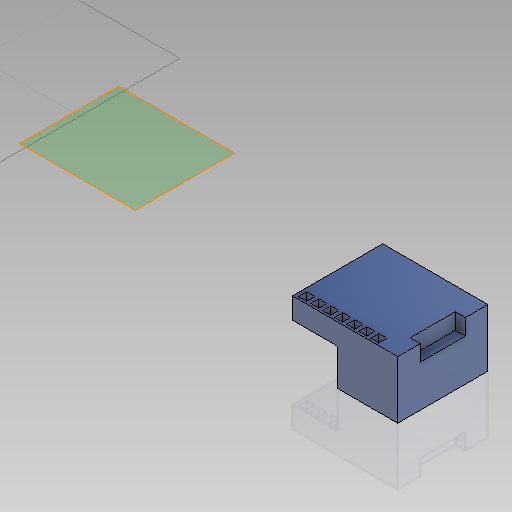
# Autodesk Inventor part: ЛЦМК0000002.00.00.00.00.04
Saved by Autodesk Inventor 2021.2 (Build 252289000, 289)
## iProperties
Created: 2025-10-23
Part Number: ЛЦМК0000002.00.00.00.00.04
Material: Типовые
Document SubType Name: Modeling
Designer: Захаров
Density: 1 g/cm^3
Appearance: С вкраплениями — сатинированная — синяя
Author: Захаров
Autodesk Inventor part; units mm, degrees
ref_plane "YZ Plane" through (0, 0, 0) normal (1, 0, 0) x (0, 1, 0)
ref_plane "XZ Plane" through (0, 0, 0) normal (0, 1, 0) x (-1, 0, 0)
ref_plane "XY Plane" through (0, 0, 0) normal (0, 0, 1) x (1, 0, 0)
ref_plane "РабПлоскость1" through (61.75, -2.8, -7.7) normal (0, -1, 0) x (1, 0, 0)
sketch "Эскиз1" plane through (61.75, -2.8, -7.7) normal (0, -1, 0) x (1, 0, 0)
  line L0 (49.15, 6.9) -> (47.55, 6.9) projected
  line L1 (47.55, 6.9) -> (47.55, 8.5) projected
  line L2 (47.55, 8.5) -> (49.15, 8.5) projected
  line L3 (49.15, 8.5) -> (49.15, 6.9) projected
  line L4 (44.35, 6.9) -> (42.75, 6.9) projected
  line L5 (42.75, 6.9) -> (42.75, 8.5) projected
  line L6 (42.75, 8.5) -> (44.35, 8.5) projected
  line L7 (44.35, 8.5) -> (44.35, 6.9) projected
  line L8 (53.95, 6.9) -> (52.35, 6.9) projected
  line L9 (52.35, 6.9) -> (52.35, 8.5) projected
  line L10 (52.35, 8.5) -> (53.95, 8.5) projected
  line L11 (53.95, 8.5) -> (53.95, 6.9) projected
  line L12 (51.55, 6.9) -> (49.95, 6.9) projected
  line L13 (49.95, 6.9) -> (49.95, 8.5) projected
  line L14 (49.95, 8.5) -> (51.55, 8.5) projected
  line L15 (51.55, 8.5) -> (51.55, 6.9) projected
  line L16 (56.35, 6.9) -> (54.75, 6.9) projected
  line L17 (54.75, 6.9) -> (54.75, 8.5) projected
  line L18 (54.75, 8.5) -> (56.35, 8.5) projected
  line L19 (56.35, 8.5) -> (56.35, 6.9) projected
  line L20 (46.75, 6.9) -> (45.15, 6.9) projected
  line L21 (45.15, 6.9) -> (45.15, 8.5) projected
  line L22 (45.15, 8.5) -> (46.75, 8.5) projected
  line L23 (46.75, 8.5) -> (46.75, 6.9) projected
  line L24 (58.75, 6.9) -> (57.15, 6.9) projected
  line L25 (57.15, 6.9) -> (57.15, 8.5) projected
  line L26 (57.15, 8.5) -> (58.75, 8.5) projected
  line L27 (58.75, 8.5) -> (58.75, 6.9) projected
  line L28 (61, 4.5) -> (63, 4.5) projected
  line L29 (63, 4.5) -> (63, 9) projected
  line L30 (63, 9) -> (42, 9) projected
  line L31 (42, 9) -> (42, -9) projected
  line L32 (42, -9) -> (63, -9) projected
  line L33 (63, -9) -> (63, -4.5) projected
  line L34 (63, -4.5) -> (61, -4.5) projected
  line L35 (61, -4.5) -> (61, 4.5) projected
  line L36 (47.55, -6.9) -> (49.15, -6.9) projected
  line L37 (49.15, -6.9) -> (49.15, -8.5) projected
  line L38 (49.15, -8.5) -> (47.55, -8.5) projected
  line L39 (47.55, -8.5) -> (47.55, -6.9) projected
  line L40 (42.75, -6.9) -> (44.35, -6.9) projected
  line L41 (44.35, -6.9) -> (44.35, -8.5) projected
  line L42 (44.35, -8.5) -> (42.75, -8.5) projected
  line L43 (42.75, -8.5) -> (42.75, -6.9) projected
  line L44 (52.35, -6.9) -> (53.95, -6.9) projected
  line L45 (53.95, -6.9) -> (53.95, -8.5) projected
  line L46 (53.95, -8.5) -> (52.35, -8.5) projected
  line L47 (52.35, -8.5) -> (52.35, -6.9) projected
  line L48 (49.95, -6.9) -> (51.55, -6.9) projected
  line L49 (51.55, -6.9) -> (51.55, -8.5) projected
  line L50 (51.55, -8.5) -> (49.95, -8.5) projected
  line L51 (49.95, -8.5) -> (49.95, -6.9) projected
  line L52 (54.75, -6.9) -> (56.35, -6.9) projected
  line L53 (56.35, -6.9) -> (56.35, -8.5) projected
  line L54 (56.35, -8.5) -> (54.75, -8.5) projected
  line L55 (54.75, -8.5) -> (54.75, -6.9) projected
  line L56 (45.15, -6.9) -> (46.75, -6.9) projected
  line L57 (46.75, -6.9) -> (46.75, -8.5) projected
  line L58 (46.75, -8.5) -> (45.15, -8.5) projected
  line L59 (45.15, -8.5) -> (45.15, -6.9) projected
  line L60 (57.15, -6.9) -> (58.75, -6.9) projected
  line L61 (58.75, -6.9) -> (58.75, -8.5) projected
  line L62 (58.75, -8.5) -> (57.15, -8.5) projected
  line L63 (57.15, -8.5) -> (57.15, -6.9) projected
  point P0 (-61.75, 7.7)
extrude "Выдавливание1" add sketch "Эскиз1" along normal blind 4.2 contours L35 L34 L33 L32 L31 L30 L29 L28 | L36 L37 L38 L39 | L40 L41 L42 L43 | L44 L45 L46 L47 | L48 L49 L50 L51 | L52 L53 L54 L55 | L56 L57 L58 L59 | L60 L61 L62 L63
sketch "Эскиз2" plane through (61.75, -7, -7.7) normal (0, -1, 0) x (1, 0, 0)
  line L0 (63, -9) -> (63, -4.5) projected
  line L1 (63, 9) -> (42, 9) projected
  line L2 (63, -9) -> (51, -9)
  line L3 (51, -9) -> (51, 9)
  line L4 (51, 9) -> (63, 9)
  line L5 (63, 9) -> (63, -9)
  point P0 (-61.75, 7.7)
  point P1 (63, -4.5)
  point P2 (63, 9)
  dimension "d2" = 12
  constraints: 8 end point, 2 parallel, 1 horizontal, 1 perpendicular, 1 point on line
  measures "d2" distance of L3.end L4.end
extrude "Выдавливание2" add sketch "Эскиз2" along normal blind 7.3
sketch "Эскиз3" plane through (61.75, -14.3, -7.7) normal (0, -1, 0) x (1, 0, 0)
  line L0 (47.55, 6.9) -> (49.15, 6.9) projected
  line L1 (49.15, 6.9) -> (49.15, 8.5) projected
  line L2 (49.15, 8.5) -> (47.55, 8.5) projected
  line L3 (47.55, 8.5) -> (47.55, 6.9) projected
  line L4 (42.75, 6.9) -> (44.35, 6.9) projected
  line L5 (44.35, 6.9) -> (44.35, 8.5) projected
  line L6 (44.35, 8.5) -> (42.75, 8.5) projected
  line L7 (42.75, 8.5) -> (42.75, 6.9) projected
  line L8 (52.35, 6.9) -> (53.95, 6.9) projected
  line L9 (53.95, 6.9) -> (53.95, 8.5) projected
  line L10 (53.95, 8.5) -> (52.35, 8.5) projected
  line L11 (52.35, 8.5) -> (52.35, 6.9) projected
  line L12 (49.95, 6.9) -> (51.55, 6.9) projected
  line L13 (51.55, 6.9) -> (51.55, 8.5) projected
  line L14 (51.55, 8.5) -> (49.95, 8.5) projected
  line L15 (49.95, 8.5) -> (49.95, 6.9) projected
  line L16 (54.75, 6.9) -> (56.35, 6.9) projected
  line L17 (56.35, 6.9) -> (56.35, 8.5) projected
  line L18 (56.35, 8.5) -> (54.75, 8.5) projected
  line L19 (54.75, 8.5) -> (54.75, 6.9) projected
  line L20 (45.15, 6.9) -> (46.75, 6.9) projected
  line L21 (46.75, 6.9) -> (46.75, 8.5) projected
  line L22 (46.75, 8.5) -> (45.15, 8.5) projected
  line L23 (45.15, 8.5) -> (45.15, 6.9) projected
  line L24 (57.15, 6.9) -> (58.75, 6.9) projected
  line L25 (58.75, 6.9) -> (58.75, 8.5) projected
  line L26 (58.75, 8.5) -> (57.15, 8.5) projected
  line L27 (57.15, 8.5) -> (57.15, 6.9) projected
  line L28 (63, 9) -> (42, 9) projected
  line L29 (63, -9) -> (63, 9) projected
  line L30 (42, -9) -> (63, -9) projected
  line L31 (42, 9) -> (42, -9) projected
  line L32 (49.15, -6.9) -> (47.55, -6.9) projected
  line L33 (47.55, -6.9) -> (47.55, -8.5) projected
  line L34 (47.55, -8.5) -> (49.15, -8.5) projected
  line L35 (49.15, -8.5) -> (49.15, -6.9) projected
  line L36 (44.35, -6.9) -> (42.75, -6.9) projected
  line L37 (42.75, -6.9) -> (42.75, -8.5) projected
  line L38 (42.75, -8.5) -> (44.35, -8.5) projected
  line L39 (44.35, -8.5) -> (44.35, -6.9) projected
  line L40 (53.95, -6.9) -> (52.35, -6.9) projected
  line L41 (52.35, -6.9) -> (52.35, -8.5) projected
  line L42 (52.35, -8.5) -> (53.95, -8.5) projected
  line L43 (53.95, -8.5) -> (53.95, -6.9) projected
  line L44 (51.55, -6.9) -> (49.95, -6.9) projected
  line L45 (49.95, -6.9) -> (49.95, -8.5) projected
  line L46 (49.95, -8.5) -> (51.55, -8.5) projected
  line L47 (51.55, -8.5) -> (51.55, -6.9) projected
  line L48 (56.35, -6.9) -> (54.75, -6.9) projected
  line L49 (54.75, -6.9) -> (54.75, -8.5) projected
  line L50 (54.75, -8.5) -> (56.35, -8.5) projected
  line L51 (56.35, -8.5) -> (56.35, -6.9) projected
  line L52 (46.75, -6.9) -> (45.15, -6.9) projected
  line L53 (45.15, -6.9) -> (45.15, -8.5) projected
  line L54 (45.15, -8.5) -> (46.75, -8.5) projected
  line L55 (46.75, -8.5) -> (46.75, -6.9) projected
  line L56 (58.75, -6.9) -> (57.15, -6.9) projected
  line L57 (57.15, -6.9) -> (57.15, -8.5) projected
  line L58 (57.15, -8.5) -> (58.75, -8.5) projected
  line L59 (58.75, -8.5) -> (58.75, -6.9) projected
  point P0 (-61.75, 7.7)
extrude "Выдавливание3" cut sketch "Эскиз3" against normal blind 7.3 contours L11 L10 L9 L8 | L15 L14 L13 L12 | L19 L18 L17 L16 | L27 L26 L25 L24
sketch "Эскиз4" plane through (61.75, -7, -7.7) normal (0, 1, 0) x (1, 0, 0)
  line L0 (61, -4.5) -> (63, -4.5) projected
  line L1 (63, 4.5) -> (63, -4.5) projected
  line L2 (63, 4.5) -> (61, 4.5) projected
  line L3 (61, 4.5) -> (61, -4.5) projected
  point P0 (-61.75, -7.7)
ref_plane "РабПлоскость2" through (10.25, -6, -12.2) normal (0, -1, 0) x (1, 0, 0)
extrude "Выдавливание4" add sketch "Эскиз4" along normal up to surface (1 mm away)
